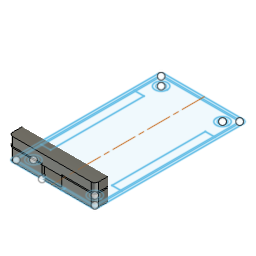
Nodemcu kotelo v7 (Autodesk Fusion 360 design; units mm, degrees)
Autodesk Fusion 360 part; units mm, degrees
note: some values were not read from the file. Chosen so that the rebuilt part matches the saved one: a side; which face or edge a step refers to. Set by a fixed rule: which sketch regions a step uses.
sketch "Top" plane through (0, 0, 0) normal (0, 0, 1) x (1, 0, 0)
  line L0 (-20.527, 30.6385) -> (9.973, 30.6385)
  line L1 (10.473, 30.1385) -> (10.473, -26.6615)
  line L2 (9.973, -27.1615) -> (-20.527, -27.1615)
  line L3 (-21.027, -26.6615) -> (-21.027, 30.1385)
  circle A0 centre (-18.027, 27.6385) radius 1.5
  circle A1 centre (-18.027, -24.1615) radius 1.5
  circle A2 centre (7.473, 27.6385) radius 1.5
  circle A3 centre (7.473, -24.1615) radius 1.5
  arc A4 (-20.527, 30.6385) -> (-21.027, 30.1385) centre (-20.527, 30.1385) ccw
  arc A5 (10.473, 30.1385) -> (9.973, 30.6385) centre (9.973, 30.1385) ccw
  arc A6 (-21.027, -26.6615) -> (-20.527, -27.1615) centre (-20.527, -26.6615) ccw
  arc A7 (9.973, -27.1615) -> (10.473, -26.6615) centre (9.973, -26.6615) ccw
  arc A8 (11.473, 30.1385) -> (9.973, 31.6385) centre (9.973, 30.1385) ccw
  line L4 (-20.527, 31.6385) -> (9.973, 31.6385)
  arc A9 (-20.527, 31.6385) -> (-22.027, 30.1385) centre (-20.527, 30.1385) ccw
  line L5 (-22.027, -26.6615) -> (-22.027, 30.1385)
  arc A10 (-22.027, -26.6615) -> (-20.527, -28.1615) centre (-20.527, -26.6615) ccw
  line L6 (9.973, -28.1615) -> (-20.527, -28.1615)
  arc A11 (9.973, -28.1615) -> (11.473, -26.6615) centre (9.973, -26.6615) ccw
  line L7 (11.473, 30.1385) -> (11.473, -26.6615)
  arc A12 (-20.527, 31.1385) -> (-21.527, 30.1385) centre (-20.527, 30.1385) ccw
  line L8 (-21.527, -26.6615) -> (-21.527, 30.1385)
  arc A13 (-21.527, -26.6615) -> (-20.527, -27.6615) centre (-20.527, -26.6615) ccw
  line L9 (9.973, -27.6615) -> (-20.527, -27.6615)
  arc A14 (9.973, -27.6615) -> (10.973, -26.6615) centre (9.973, -26.6615) ccw
  line L10 (10.973, 30.1385) -> (10.973, -26.6615)
  arc A15 (10.973, 30.1385) -> (9.973, 31.1385) centre (9.973, 30.1385) ccw
  line L11 (-20.527, 31.1385) -> (9.973, 31.1385)
  circle A16 centre (-18.027, 27.6385) radius 2.5
  circle A17 centre (7.473, 27.6385) radius 2.5
  circle A18 centre (-18.027, -24.1615) radius 2.5
  circle A19 centre (7.473, -24.1615) radius 2.5
  point P0 (-21.027, 30.6385)
  point P1 (10.473, 30.6385)
  point P2 (-21.027, -27.1615)
  dimension "d1" = 31.5
  dimension "d4" = 57.8
  dimension "d5" = 3
  dimension "d6" = 0.5
  dimension "d7" = 0.5
  dimension "d8" = 0.5
  dimension "d9" = 0.5
  dimension "d11" = -1
  dimension "d29" = 3
  dimension "d30" = 3
  dimension "d33" = 3
  dimension "d34" = 3
  dimension "d35" = 3
  dimension "d36" = 3
  dimension "d37" = 3
  dimension "d38" = 3
  dimension "d48" = -0.5
  dimension "d49" = 1
  dimension "d50" = 1
  dimension "d51" = 1
  dimension "d52" = 1
  dimension "d53" = 25.5
  constraint horizontal L0
  constraint vertical L1
  constraint horizontal L2
  constraint vertical L3
  constraint coincident P0 L0
  constraint coincident P0 L3
  constraint tangent L0 A4
  constraint tangent L3 A4
  constraint coincident P1 L0
  constraint coincident P1 L1
  constraint tangent L0 A5
  constraint tangent L1 A5
  constraint coincident P2 L2
  constraint coincident P2 L3
  constraint tangent L2 A6
  constraint tangent L3 A6
  constraint tangent L1 A7
  constraint tangent L2 A7
  measures "d1" distance of P0 P1
  measures "d4" distance of P0 P2
  measures "d5" diameter of A0
  measures "d6" radius of A4
  measures "d7" radius of A5
  measures "d8" radius of A6
  measures "d9" radius of A7
  measures "d11" distance of A5
  measures "d29" distance of L0 A0.centre
  measures "d30" distance of L3 A0.centre
  measures "d33" distance of L1 A2.centre
  measures "d34" distance of L0 A2.centre
  measures "d35" distance of L1 A3.centre
  measures "d36" distance of L2 A3.centre
  measures "d37" distance of L2 A1.centre
  measures "d38" distance of L3 A1.centre
  measures "d48" distance of A4
  measures "d53" distance of A0.centre A2.centre
extrude "Extrude1" add sketch "Top" along normal blind 5 contours A8 L4 A9 L5 A10 L6 A11 L7 | A12 L8 A13 L9 A14 L10 A15 L11 makes body 1
extrude "Extrude2" add sketch "Top" along normal blind 5 separate body contours A0 | A1 | A2 | A3 makes body 2 at (5.9804, 27.4892, 3.3333) makes body 3 at (-16.5289, -24.2362, 3.3333) makes body 4 at (-16.5289, 27.5638, 3.3333) makes body 5 at (5.9804, -24.3108, 3.3333)
extrude "Extrude3" add sketch "Top" along normal blind 1 contours L0 L1 L2 L3 A4 A5 A6 A7 | A12 L8 A13 L9 A14 L10 A15 L11 | A16 | A17 | A18 | A19 bodies 1 2 3 4 5
sketch "Front" plane through (0, -28.1615, 0) normal (0, -1, 0) x (1, 0, 0)
  line L0 (-20.527, 0) -> (9.973, 0)
  line L1 (9.973, 0) -> (9.973, 5)
  line L2 (9.973, 5) -> (-20.527, 5)
  line L3 (-20.527, 5) -> (-20.527, 0)
  line L4 (-8.777, 4) -> (-1.777, 4)
  line L5 (-1.277, 3.5) -> (-1.277, 1.5)
  line L6 (-1.777, 1) -> (-8.777, 1)
  line L7 (-9.277, 1.5) -> (-9.277, 3.5)
  arc A0 (-8.777, 4) -> (-9.277, 3.5) centre (-8.777, 3.5) ccw
  arc A1 (-1.277, 3.5) -> (-1.777, 4) centre (-1.777, 3.5) ccw
  arc A2 (-9.277, 1.5) -> (-8.777, 1) centre (-8.777, 1.5) ccw
  arc A3 (-1.777, 1) -> (-1.277, 1.5) centre (-1.777, 1.5) ccw
  line L8 (-9.277, 3.5) -> (-9.277, 5)
  line L9 (-1.277, 3.5) -> (-1.277, 5)
  point P0 (-9.277, 4)
  point P1 (-1.277, 4)
  point P2 (-9.277, 1)
  dimension "d40" = 8
  dimension "d41" = 3
  dimension "d42" = 0.5
  dimension "d43" = 0.5
  dimension "d44" = 0.5
  dimension "d45" = 0.5
  constraint horizontal L4
  constraint vertical L5
  constraint horizontal L6
  constraint vertical L7
  constraint coincident P0 L4
  constraint coincident P0 L7
  constraint tangent L4 A0
  constraint tangent L7 A0
  constraint coincident P1 L4
  constraint coincident P1 L5
  constraint tangent L4 A1
  constraint tangent L5 A1
  constraint coincident P2 L6
  constraint coincident P2 L7
  constraint tangent L6 A2
  constraint tangent L7 A2
  constraint tangent L5 A3
  constraint tangent L6 A3
  constraint coincident L2 L8.end
  constraint tangent A0 L8
  constraint coincident L2 L9.end
  constraint tangent A1 L9
  measures "d40" distance of P0 P1
  measures "d41" distance of P0 P2
  measures "d42" radius of A0
  measures "d43" radius of A1
  measures "d44" radius of A2
  measures "d45" radius of A3
extrude "Extrude6" cut sketch "Front" against normal up to surface (1 mm away) contours L2 L4 A0 A1 L8 L9 | L4 L5 L6 L7 A0 A1 A2 A3 bodies 1
sketch "Topv2" plane through (0, 0, 0) normal (0, 0, 1) x (1, 0, 0)
  circle A0 centre (-20.0134, 24.6) radius 1.5
  circle A1 centre (-20.0134, 24.6) radius 2.5
  circle A2 centre (4.9866, 24.6) radius 2.5
  circle A3 centre (4.9866, 24.6) radius 1.5
  circle A4 centre (-20, 76.6) radius 2.5
  circle A5 centre (-20, 76.6) radius 1.5
  circle A6 centre (5, 76.6) radius 1.5
  circle A7 centre (5, 76.6) radius 2.5
  line L0 (8.5, 20.6) -> (-23.5, 20.6)
  line L1 (-24, 21.1) -> (-24, 80.1)
  line L2 (-23.5, 80.6) -> (8.5, 80.6)
  line L3 (9, 80.1) -> (9, 21.1)
  arc A8 (9, 80.1) -> (8.5, 80.6) centre (8.5, 80.1) ccw
  arc A9 (-23.5, 80.6) -> (-24, 80.1) centre (-23.5, 80.1) ccw
  arc A10 (-24, 21.1) -> (-23.5, 20.6) centre (-23.5, 21.1) ccw
  arc A11 (8.5, 20.6) -> (9, 21.1) centre (8.5, 21.1) ccw
  arc A12 (8.5, 19.6) -> (10, 21.1) centre (8.5, 21.1) ccw
  line L4 (10, 80.1) -> (10, 21.1)
  arc A13 (10, 80.1) -> (8.5, 81.6) centre (8.5, 80.1) ccw
  line L5 (-23.5, 81.6) -> (8.5, 81.6)
  arc A14 (-23.5, 81.6) -> (-25, 80.1) centre (-23.5, 80.1) ccw
  line L6 (-25, 21.1) -> (-25, 80.1)
  arc A15 (-25, 21.1) -> (-23.5, 19.6) centre (-23.5, 21.1) ccw
  line L7 (8.5, 19.6) -> (-23.5, 19.6)
  line L8 (-7.5, 81.6) -> (-7.5, 19.6)
  line L9 (-3.5, 20.6) -> (-3.5, 19.6)
  line L10 (-11.5, 20.6) -> (-11.5, 19.6)
  line L11 (-23.5, 21.1) -> (-23.5, 80.1)
  line L12 (8.5, 21.1) -> (-23.5, 21.1)
  line L13 (8.5, 80.1) -> (8.5, 21.1)
  line L14 (-23.5, 80.1) -> (8.5, 80.1)
  line L15 (-20, 69.6) -> (-20, 31.6)
  line L16 (5, 69.6) -> (5, 31.6)
  line L17 (-24, 69.6) -> (-20, 69.6)
  line L18 (5, 69.6) -> (9, 69.6)
  line L19 (-24, 31.6) -> (-20, 31.6)
  line L20 (5, 31.6) -> (9, 31.6)
  line L21 (-3.5, 20.6) -> (-3.5, 21.1)
  line L22 (-11.5, 20.6) -> (-11.5, 21.1)
  dimension "d54" = 3
  dimension "d55" = 1
  dimension "d56" = 1
  dimension "d57" = 3
  dimension "d58" = 25
  dimension "d59" = 1
  dimension "d60" = 3
  dimension "d61" = 52
  dimension "d62" = 1
  dimension "d63" = 3
  dimension "d64" = 52
  dimension "d65" = 25
  dimension "d67" = 0.5
  dimension "d68" = 0.5
  dimension "d69" = 0.5
  dimension "d70" = 0.5
  dimension "d71" = -1
  dimension "d73" = 8
  dimension "d86" = 59
  dimension "d87" = 32
  dimension "d88" = 0.5
  dimension "d89" = 11
  dimension "d90" = 11
  dimension "d91" = 4
  dimension "d92" = 4
  dimension "d93" = 11
  dimension "d94" = 11
  constraint tangent L2 A8
  constraint tangent L3 A8
  constraint tangent L1 A9
  constraint tangent L2 A9
  constraint tangent L0 A10
  constraint tangent L1 A10
  constraint tangent L0 A11
  constraint tangent L3 A11
  constraint midpoint L5 L8.start
  constraint midpoint L7 L8.end
  constraint perpendicular L7 L8
  constraint coincident L0 L9.start
  constraint perpendicular L0 L9
  constraint coincident L7 L9.end
  constraint symmetric L8 L9.start L10.start
  constraint symmetric L8 L9.end L10.end
  constraint coincident L1 L17.start
  constraint coincident L3 L18.end
  constraint perpendicular L3 L17
  constraint coincident L1 L19.start
  constraint coincident L3 L20.end
  constraint perpendicular L3 L19
  constraint perpendicular L15 L19
  constraint coincident L16.start L17
  constraint coincident L16.end L19
  constraint perpendicular L16 L19
  constraint collinear L17 L18
  constraint collinear L19 L20
  constraint coincident L12 L21.end
  constraint perpendicular L12 L21
  constraint coincident L12 L22.end
  constraint perpendicular L12 L22
  measures "d54" diameter of A0
  measures "d57" diameter of A3
  measures "d58" distance of A0.centre A2.centre
  measures "d60" diameter of A5
  measures "d61" distance of A0.centre A4.centre
  measures "d63" diameter of A6
  measures "d64" distance of A2.centre A6.centre
  measures "d65" distance of A4.centre A6.centre
  measures "d67" radius of A8
  measures "d68" radius of A9
  measures "d69" radius of A10
  measures "d70" radius of A11
  measures "d71" distance of A11
  measures "d73" distance of L9 L10
  measures "d86" distance of L1.end L1.start
  measures "d87" distance of L2.end L2.start
  measures "d89" distance of L2 L17
  measures "d90" distance of L0 L19
  measures "d91" distance of L1 L15
  measures "d92" distance of L3 L16
  measures "d93" distance of L2 L18
  measures "d94" distance of L0 L20
extrude "Extrude7" add sketch "Topv2" along normal blind 8 separate body contours A0 | A3 | A5 | A6 makes body 6 at (-18.6178, 77.1827, 5.3333) makes body 7 at (6.3822, 77.1827, 5.3333) makes body 8 at (-21.506, 24.4506, 5.3333) makes body 9 at (6.4847, 24.5252, 5.3333)
extrude "Extrude8" add sketch "Topv2" along normal blind 3 contours A1 | A2 | A4 | A7 bodies 6 7 8 9
extrude "Extrude9" add sketch "Topv2" along normal blind 5 separate body contours L0 L2 L3 A8 A11 A12 L4 A13 L5 L7 L8 L9 | L0 L1 L2 A9 A10 L5 A14 L6 A15 L7 L8 L10 makes body 10
extrude "Extrude10" add sketch "Topv2" along normal blind 1 contours L0 L3 A11 L12 L13 L20 L21 | L0 L7 L8 L9 | L0 L8 L12 L21 | L0 L7 L8 L10 | L0 L8 L12 L22 | L8 L12 L13 L14 L16 L18 L20 | L3 L13 L18 L20 | L0 L1 A10 L11 L12 L19 L22 | L8 L11 L12 L14 L15 L17 L19 | L2 L3 A8 L8 L13 L14 L18 | L13 L16 L18 L20 | L1 L2 A9 L8 L11 L14 L17 | L1 L11 L17 L19 | L11 L15 L17 L19 bodies 6 7 8 9 10
fillet "Fillet1" radius 0.5 1 edges at (-11.5, 20.1, 1) on bodies 6
fillet "Fillet2" radius 0.5 1 edges at (-3.5, 20.1, 1) on bodies 6
extrude "Extrude11" add sketch "Topv2" along normal blind 1 from surface at 8 separate body contours A0 | A1 | A2 | A3 | A4 | A5 | A6 | A7 | L0 L2 L3 A8 A11 A12 L4 A13 L5 L7 L8 L9 | L0 L3 A11 L12 L13 L20 L21 | L0 L7 L8 L9 | L0 L8 L12 L21 | L0 L7 L8 L10 | L0 L8 L12 L22 | L8 L12 L13 L14 L16 L18 L20 | L3 L13 L18 L20 | L0 L1 L2 A9 A10 L5 A14 L6 A15 L7 L8 L10 | L0 L1 A10 L11 L12 L19 L22 | L8 L11 L12 L14 L15 L17 L19 | L2 L3 A8 L8 L13 L14 L18 | L13 L16 L18 L20 | L1 L2 A9 L8 L11 L14 L17 | L1 L11 L17 L19 | L11 L15 L17 L19 makes body 11
extrude "Extrude12" cut sketch "Topv2" along normal up to surface (1 mm away) from surface at 8 contours L13 L16 L18 L20 | L11 L15 L17 L19 bodies 11
extrude "Extrude13" add sketch "Topv2" along normal up to surface (2.5 mm away) from surface at 5.5 contours L0 L2 L3 A8 A11 A12 L4 A13 L5 L7 L8 L9 | L0 L1 L2 A9 A10 L5 A14 L6 A15 L7 L8 L10 bodies 11
extrude "Extrude14" add sketch "Topv2" against normal blind 4 from surface at 8 contours L0 L3 A11 L12 L13 L20 L21 | L0 L8 L12 L21 | L0 L8 L12 L22 | L3 L13 L18 L20 | L0 L1 A10 L11 L12 L19 L22 | L2 L3 A8 L8 L13 L14 L18 | L1 L2 A9 L8 L11 L14 L17 | L1 L11 L17 L19 bodies 11
extrude "Extrude15" add sketch "Topv2" against normal blind 2 from surface at 8 contours A1 | A2 | A4 | A7 bodies 11
extrude "Extrude16" add sketch "Topv2" against normal up to surface (2.5 mm away) from surface at 8 contours L0 L7 L8 L9 | L0 L7 L8 L10 bodies 11
extrude "Extrude17" add sketch "Topv2" against normal up to surface (0.5 mm away) from surface at 5.5 contours L0 L7 L8 L9 | L0 L7 L8 L10 bodies 11
extrude "Extrude18" cut sketch "Topv2" along normal up to surface (1 mm away) from surface at 4 contours L0 L8 L12 L21 | L0 L8 L12 L22 bodies 11
extrude "Extrude19" cut 4 faces at (-19.573, 25.246, 8) (-19.8613, 77.7712, 8) (4.916, 77.7203, 8) (5.3256, 25.3552, 8) along direction (0, 0, -1) blind 3 on bodies 6 bodies 6
hidden bodies 1
equation "d1 = nodemcuWidth + 0.5 mm"
equation "nodemcuWidth = 31 mm"
equation "nodemcuHeight = 57.3 mm"
equation "d4 = nodemcuHeight + 0.5 mm"
equation "d6 = nodemcuCornerRadius"
equation "d7 = nodemcuCornerRadius"
equation "d8 = nodemcuCornerRadius"
equation "d9 = nodemcuCornerRadius"
equation "nodemcuCornerRadius = 0.5 mm"
equation "d12 = 5 mm"
equation "d14 = d12"
equation "powerSocketRadius = 0.5 mm"
equation "d30 = d29"
equation "d33 = d29"
equation "d34 = d29"
equation "d35 = d29"
equation "d36 = d29"
equation "d37 = d29"
equation "d38 = d29"
equation "d42 = powerSocketRadius"
equation "d43 = powerSocketRadius"
equation "d44 = powerSocketRadius"
equation "d45 = powerSocketRadius"
equation "d64 = d61"
equation "d65 = d58"
equation "d67 = nodemcuCornerRadius"
equation "d68 = nodemcuCornerRadius"
equation "d69 = nodemcuCornerRadius"
equation "d70 = nodemcuCornerRadius"
equation "d83 = powerSocketRadius"
equation "d85 = powerSocketRadius"
named bodies: "Base", "Basev2", "Top"
